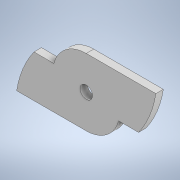
# Autodesk Inventor part: ArmaPrime
Saved by Autodesk Inventor 2022 (Build 260153000, 153)
## iProperties
Created: 2021-04-12
Part Number: ArmaPrime
Material: Genérico
Document SubType Name: Modeling
Designer: dcast
Density: 1 g/cm^3
Appearance: Valor por defecto
Author: dcast
Autodesk Inventor part; units mm, degrees
ref_plane "YZ Plane" through (0, 0, 0) normal (1, 0, 0) x (0, 1, 0)
ref_plane "XZ Plane" through (0, 0, 0) normal (0, 1, 0) x (-1, 0, 0)
ref_plane "XY Plane" through (0, 0, 0) normal (0, 0, 1) x (1, 0, 0)
sketch "Sketch3" plane through (0, 0, 0) normal (0, 0, 1) x (1, 0, 0)
  line L0 (13.0384, -3.5) -> (21.0384, -3.5)
  line L1 (-13.0384, 3.5) -> (-21.0384, 3.5)
  line L2 (0, 13.5) -> (28, 13.5)
  line L3 (0, -13.5) -> (-28, -13.5)
  arc A0 (-21.0384, 3.5) -> (-28, -13.5) centre (11.5082, -19.7534) ccw
  arc A1 (21.0384, -3.5) -> (28, 13.5) centre (-11.5082, 19.7534) ccw
  arc A2 (0, 13.5) -> (-13.0384, 3.5) centre (0, 0) ccw
  arc A3 (0, -13.5) -> (13.0384, -3.5) centre (0, 0) ccw
  circle A4 centre (0, 0) radius 2.5
  dimension "d29" = 8
  dimension "d30" = 8
  dimension "d33" = 28
  dimension "d34" = 28
  dimension "d35" = 40
  dimension "d36" = 40
  dimension "d37" = 5
  constraints: 8 end point, 8 point on circle, 5 centre point, 4 horizontal, 2 coincident, 2 tangent
  measures "d29" distance of L0.start L0.end
  measures "d30" distance of L1.start L1.end
  measures "d33" distance of L2.start L2.end
  measures "d34" distance of L3.start L3.end
  measures "d35" radius of A0
  measures "d36" radius of A1
  measures "d37" diameter of A4
extrude "Extrusion2" add sketch "Sketch3" along normal blind 3
body "Solid2"
